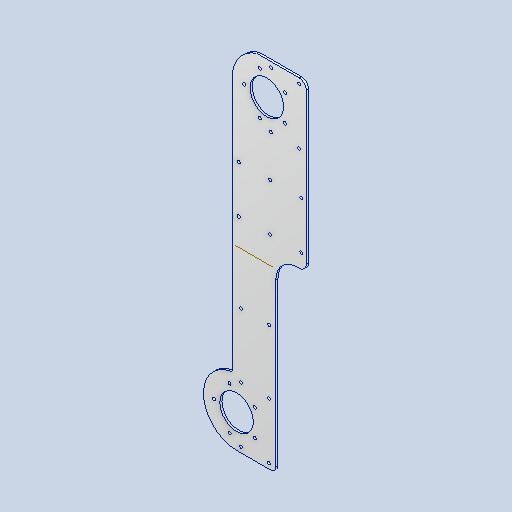
# Autodesk Inventor part: blacha
Saved by Autodesk Inventor 2023 (Build 270158000, 158)
## iProperties
Created: 2023-01-20
Part Number: blacha
Material: Aluminum 6061
Document SubType Name: Modeling
Designer: Kamil
Density: 2.7 g/cm^3
Appearance: Aluminum - Flat
Mass: 107.528 g
Surface Area: 763.261 cm^2
Volume: 107.528 cm^3
Author: Kamil
Autodesk Inventor part; units mm, degrees
ref_plane "YZ Plane" through (0, 0, 0) normal (1, 0, 0) x (0, 1, 0)
ref_plane "XZ Plane" through (0, 0, 0) normal (0, 1, 0) x (-1, 0, 0)
ref_plane "XY Plane" through (0, 0, 0) normal (0, 0, 1) x (1, 0, 0)
sketch "Sketch1" plane through (0, 0, 0) normal (0, 0, 1) x (1, 0, 0)
  circle A0 centre (-40, 69.5) radius 2 projected
  arc A1 (-40, 77) -> (-46, 74) centre (-40, 69.5) ccw projected
  line L0 (-30, 77) -> (-40, 77) projected
  line L1 (-30, 73) -> (-30, 77) projected
  line L2 (-34, 73) -> (-30, 73) projected
  line L3 (-34, 66) -> (-34, 73) projected
  line L4 (-30, 66) -> (-34, 66) projected
  line L5 (-30, 62) -> (-30, 66) projected
  line L6 (-30, 62) -> (-40, 62) projected
  arc A2 (-46, 65) -> (-40, 62) centre (-40, 69.5) ccw projected
  line L7 (-46, 74) -> (-46, 65) projected
  arc A3 (0, 74) -> (-6, 77) centre (-6, 69.5) ccw projected
  line L8 (0, 74) -> (0, 65) projected
  arc A4 (-6, 62) -> (0, 65) centre (-6, 69.5) ccw projected
  line L9 (-6, 62) -> (-16, 62) projected
  line L10 (-16, 66) -> (-16, 62) projected
  line L11 (-12, 66) -> (-16, 66) projected
  line L12 (-12, 73) -> (-12, 66) projected
  line L13 (-16, 73) -> (-12, 73) projected
  line L14 (-16, 77) -> (-16, 73) projected
  line L15 (-6, 77) -> (-16, 77) projected
  circle A5 centre (-6, 69.5) radius 2 projected
  circle A6 centre (-43.375, 22.1232) radius 2 projected
  circle A7 centre (-53.625, 22.1232) radius 2 projected
  circle A8 centre (-38.25, 31) radius 2 projected
  circle A9 centre (-58.75, 31) radius 2 projected
  circle A10 centre (-43.375, 39.8768) radius 2 projected
  arc A11 (-46.014, 25.5393) -> (-48.9684, 25.0183) centre (-48.5, 31) ccw projected
  line L16 (-48.76, 23.8365) -> (-48.9684, 25.0183) projected
  line L17 (-45.8056, 24.3575) -> (-48.76, 23.8365) projected
  line L18 (-46.014, 25.5393) -> (-45.8056, 24.3575) projected
  circle A12 centre (-53.625, 39.8768) radius 2 projected
  circle A13 centre (-48.5, 31) radius 13.4542 projected
  circle A14 centre (-40, -7.5) radius 2 projected
  arc A15 (-40, 0) -> (-46, -3) centre (-40, -7.5) ccw projected
  line L19 (-30, 0) -> (-40, 0) projected
  line L20 (-30, -4) -> (-30, 0) projected
  line L21 (-34, -4) -> (-30, -4) projected
  line L22 (-34, -11) -> (-34, -4) projected
  line L23 (-30, -11) -> (-34, -11) projected
  line L24 (-30, -15) -> (-30, -11) projected
  line L25 (-30, -15) -> (-40, -15) projected
  arc A16 (-46, -12) -> (-40, -15) centre (-40, -7.5) ccw projected
  line L26 (-46, -3) -> (-46, -12) projected
  arc A17 (0, -3) -> (-6, 0) centre (-6, -7.5) ccw projected
  line L27 (0, -3) -> (0, -12) projected
  arc A18 (-6, -15) -> (0, -12) centre (-6, -7.5) ccw projected
  line L28 (-6, -15) -> (-16, -15) projected
  line L29 (-16, -11) -> (-16, -15) projected
  line L30 (-12, -11) -> (-16, -11) projected
  line L31 (-12, -4) -> (-12, -11) projected
  line L32 (-16, -4) -> (-12, -4) projected
  line L33 (-16, 0) -> (-16, -4) projected
  line L34 (-6, 0) -> (-16, 0) projected
  circle A19 centre (-6, -7.5) radius 2 projected
  circle A20 centre (-48.5, 31) radius 27.5 projected
  circle A21 centre (-48.5, 31) radius 24.5
  circle A22 centre (-48.5, 31) radius 19.1667 projected
  circle A23 centre (-48.5, 31) radius 23.3333 projected
  line L35 (-40, -15) -> (-69.5534, -15)
  circle A24 centre (-48.5, 31) radius 46
  line L36 (0, 77) -> (-48.5, 77)
  line L37 (-48.5, 77) -> (-48.5, -15)
  line L38 (-48.5, -15) -> (0, -15)
  line L39 (0, -15) -> (0, 77)
  point P0 (0, 0)
  point P1 (-14.5147, 62)
  point P2 (-16, 63.5538)
  point P3 (-14.5147, 0)
  point P4 (-16, -1.5538)
  point P5 (0, 74)
  point P6 (-6, 77)
  point P7 (-42.4251, 76.5971)
  point P8 (-42.4251, -14.5971)
  point P9 (0, -3)
  constraints: 10 end point, 3 horizontal, 2 parallel, 1 centre point, 1 coincident, 1 perpendicular, 1 point on circle, 1 point on line, 1 tangent, 4 other
extrude "Extrusion1" add sketch "Sketch1" against normal blind 3 contours L0 L1 A24 A1 | A24 L1 L2 L3 L4 L5 L6 A2 L7 A1 | A1 L7 A2 L6 L5 L4 L3 L2 L1 A24 L10 L9 L34 L33 L24 L23 L22 L21 L20 L19 A15 L26 A16 L37 A20 | L36 L14 L13 L12 L11 L10 A24 L1 | L37 A20 A24 | L15 A3 L8 A4 L9 A24 L10 L11 L12 L13 L14 | L37 A21 A20 | A20 L37 A21 | L36 L39 A3 | A16 A24 L24 L25 | A16 L26 A15 L19 L20 L21 L22 L23 L24 A24 | L37 A23 A21 | A21 L37 A23 | L9 A4 L39 A17 L34 A24 | L24 A24 L33 L32 L31 L30 L29 L38 | L29 L30 L31 L32 L33 A24 L34 A17 L27 A18 L28 | A18 L39 L38
sketch "Sketch2" plane through (0, 0, 0) normal (0, 0, 1) x (1, 0, 0)
  line L0 (0, 77) -> (-40, 77) projected
  arc A0 (-40, 77) -> (-42.4251, 76.5971) centre (-40, 69.5) ccw projected
  arc A1 (-42.4251, 76.5971) -> (-42.4251, -14.5971) centre (-48.5, 31) ccw projected
  arc A2 (-42.4251, -14.5971) -> (-40, -15) centre (-40, -7.5) ccw projected
  line L1 (-40, -15) -> (0, -15) projected
  line L2 (0, -15) -> (0, 77) projected
  circle A3 centre (-6, -7.5) radius 2 projected
  line L3 (-14.5147, 62) -> (-16, 62) projected
  line L4 (-16, 62) -> (-16, 63.5538) projected
  arc A4 (-14.5147, 62) -> (-16, 63.5538) centre (-48.5, 31) ccw projected
  circle A5 centre (-6, 69.5) radius 2 projected
  circle A6 centre (-40, -7.5) radius 2 projected
  circle A7 centre (-48.5, 31) radius 23.3333 projected
  circle A8 centre (-40, 69.5) radius 2 projected
  arc A9 (-16, -1.5538) -> (-14.5147, 0) centre (-48.5, 31) ccw projected
  line L5 (-16, -1.5538) -> (-16, 0) projected
  line L6 (-16, 0) -> (-14.5147, 0) projected
  point P0 (0, 0)
extrude "Extrusion2" add sketch "Sketch2" along normal blind 3
extrude "Extrusion3" cut sketch "Sketch2" against normal blind 3
sketch "Sketch3" plane through (0, 0, 3) normal (0, 0, 1) x (1, 0, 0)
  arc A0 (-40, 77) -> (-42.4251, 76.5971) centre (-40, 69.5) ccw projected
  arc A1 (-42.4251, 76.5971) -> (-42.4251, -14.5971) centre (-48.5, 31) ccw projected
  arc A2 (-42.4251, -14.5971) -> (-40, -15) centre (-40, -7.5) ccw projected
  line L0 (-40, -15) -> (0, -15) projected
  line L1 (0, -15) -> (0, 77) projected
  line L2 (0, 77) -> (-40, 77) projected
  circle A3 centre (-6, -7.5) radius 2 projected
  circle A4 centre (-6, 69.5) radius 2 projected
  circle A5 centre (-40, -7.5) radius 2 projected
  circle A6 centre (-40, 69.5) radius 2 projected
  line L3 (-16, 0) -> (-14.5147, 0) projected
  arc A7 (-16, -1.5538) -> (-14.5147, 0) centre (-48.5, 31) ccw projected
  line L4 (-16, -1.5538) -> (-16, 0) projected
  circle A8 centre (-48.5, 31) radius 23.3333 projected
  line L5 (-14.5147, 62) -> (-16, 62) projected
  line L6 (-16, 62) -> (-16, 63.5538) projected
  arc A9 (-14.5147, 62) -> (-16, 63.5538) centre (-48.5, 31) ccw projected
  line L7 (0, -15) -> (0, 77) projected
  arc A10 (-42.4251, 76.5971) -> (-42.4251, -14.5971) centre (-48.5, 31) ccw projected
  line L8 (0, -15) -> (-48.5, -15)
  line L9 (-48.5, -15) -> (-48.5, 31)
  line L10 (-48.5, 31) -> (0, 31)
  line L11 (0, 31) -> (0, -15)
  line L12 (0, 77) -> (-40, 77) projected
  line L13 (0, 77) -> (-48.5, 77)
  line L14 (-48.5, 77) -> (-48.5, 31)
  line L15 (-48.5, 31) -> (0, 31)
  line L16 (0, 31) -> (0, 77)
  line L17 (-7, 271.4196) -> (-7, 337.7)
  line L18 (-39, 271.4196) -> (-39, 337.7)
  line L19 (-48.5, -15) -> (0, -15)
  line L20 (0, -15) -> (0, 420.1653)
  line L21 (0, 420.1653) -> (-48.5, 420.1653)
  line L22 (-48.5, 420.1653) -> (-48.5, -15)
  circle A11 centre (-24.25, 395.9153) radius 24.25
  point P0 (0, 0)
  point P1 (-40, -15)
  point P2 (-48.5, 395.9153)
  point P3 (0, 77)
  point P4 (0, 395.9153)
  constraints: 28 end point, 6 parallel, 3 horizontal, 3 perpendicular, 3 tangent, 2 vertical, 1 centre point, 4 other
extrude "Extrusion4" add sketch "Sketch3" against normal up to surface (3 mm away) contours L13 L22 A11 L20 L2 | A0 A1 L13 | A11 | A1 A2 L8 | L3 A7 L4 | L5 L6 A9
sketch "Sketch4" plane through (0, 0, 3) normal (0, 0, 1) x (1, 0, 0)
  arc A0 (-30.4833, -4.1518) -> (-30.4833, 66.1518) centre (-48.5, 31) ccw projected
  arc A1 (-50.0418, 70.4699) -> (-50.0418, -8.4699) centre (-48.5, 31) ccw projected
  circle A2 centre (-48.5, 31) radius 23.3333 projected
  arc A3 (-50.0418, -8.4699) -> (-43.2432, -5.1587) centre (-49.7295, -0.476) ccw projected
  arc A4 (-38.0441, -4.0108) -> (-43.2432, -5.1587) centre (-40, -7.5) ccw projected
  arc A5 (-38.0441, -4.0108) -> (-30.4833, -4.1518) centre (-34.1323, 2.9676) ccw projected
  arc A6 (-30.4833, 66.1518) -> (-38.0441, 66.0108) centre (-34.1323, 59.0324) ccw projected
  arc A7 (-43.2432, 67.1587) -> (-38.0441, 66.0108) centre (-40, 69.5) ccw projected
  arc A8 (-43.2432, 67.1587) -> (-50.0418, 70.4699) centre (-49.7295, 62.476) ccw projected
  circle A9 centre (-23.0834, 49.4663) radius 3.75 projected
  circle A10 centre (-58.2083, 1.121) radius 3.75 projected
  circle A11 centre (-79.9167, 31) radius 3.75 projected
  circle A12 centre (-23.0834, 12.5337) radius 3.75 projected
  circle A13 centre (-58.2083, 60.879) radius 3.75 projected
  point P0 (0, 0)
  point P1 (-48.5, 31)
  point P2 (-48.5, 31)
  point P3 (-48.5, 31)
  point P4 (-48.5, 31)
extrude "Extrusion5" [suppressed]
sketch "Sketch5" plane through (0, 0, 3) normal (0, 0, 1) x (1, 0, 0)
  circle A0 centre (-23.0834, 49.4663) radius 2.1 projected
  circle A1 centre (-23.0834, 12.5337) radius 2.1 projected
  circle A2 centre (-40, -7.5) radius 2 projected
  circle A3 centre (-58.2083, 1.121) radius 2.1 projected
  circle A4 centre (-79.9167, 31) radius 2.1 projected
  circle A5 centre (-58.2083, 60.879) radius 2.1 projected
  point P0 (0, 0)
extrude "Extrusion6" cut sketch "Sketch5" against normal through all contours A0 | A1 | A3 | A4 | A5
sketch "Sketch6" plane through (0, 0, 3) normal (0, 0, 1) x (1, 0, 0)
  circle A0 centre (-58.2083, 1.121) radius 2.1 projected
  circle A1 centre (-79.9167, 31) radius 2.1 projected
  circle A2 centre (-23.0834, 12.5337) radius 2.1 projected
  circle A3 centre (-58.2083, 60.879) radius 2.1 projected
  circle A4 centre (-23.0834, 49.4663) radius 2.1 projected
  arc A5 (-48.5, 77) -> (-48.5, -15) centre (-48.5, 31) ccw projected
  line L0 (-48.5, -15) -> (0, -15) projected
  line L1 (0, -15) -> (0, 395.9153) projected
  arc A6 (0, 395.9153) -> (-48.5, 395.9153) centre (-24.25, 395.9153) ccw projected
  line L2 (-48.5, 395.9153) -> (-48.5, 77) projected
  circle A7 centre (-6, -7.5) radius 2 projected
  circle A8 centre (-6, 69.5) radius 2 projected
  circle A9 centre (-40, -7.5) radius 2 projected
  circle A10 centre (-40, 69.5) radius 2 projected
  circle A11 centre (-48.5, 31) radius 23.3333 projected
  arc A12 (-6, 135.8558) -> (0, 138.8558) centre (-6, 143.3558) ccw projected
  line L3 (-40, 135.8558) -> (-6, 135.8558) projected
  arc A13 (-46, 138.8558) -> (-40, 135.8558) centre (-40, 143.3558) ccw projected
  line L4 (-46, 138.8558) -> (-46, 147.8558) projected
  arc A14 (-40, 150.8558) -> (-46, 147.8558) centre (-40, 143.3558) ccw projected
  line L5 (-40, 150.8558) -> (-6, 150.8558) projected
  arc A15 (0, 147.8558) -> (-6, 150.8558) centre (-6, 143.3558) ccw projected
  line L6 (0, 138.8558) -> (0, 147.8558) projected
  circle A16 centre (-40, 143.3558) radius 2 projected
  circle A17 centre (-6, 143.3558) radius 2 projected
  point P0 (0, 0)
extrude "Extrusion7" cut sketch "Sketch6" against normal blind 10 contours A16 | A17
sketch "Sketch7" plane through (0, 0, 3) normal (0, 0, 1) x (1, 0, 0)
  arc A0 (-6, -15) -> (0, -12) centre (-6, -7.5) ccw
  line L0 (0, -15) -> (0, 395.9153) projected
  line L1 (-48.5, -15) -> (0, -15) projected
  point P0 (0, 0)
  constraints: 2 point on circle, 1 centre point, 4 other
extrude "Extrusion8" cut sketch "Sketch7" against normal through all
sketch "Sketch8" plane through (0, 0, 3) normal (0, 0, 1) x (1, 0, 0)
  arc A0 (-4, 323.7734) -> (-4, 343.7734) centre (-4, 333.7734) ccw
  arc A1 (-4, 258.1618) -> (-4, 278.1618) centre (-4, 268.1618) ccw
  arc A2 (-42, 278.1618) -> (-42, 258.1618) centre (-42, 268.1618) ccw
  arc A3 (-42, 343.7734) -> (-42, 323.7734) centre (-42, 333.7734) ccw
  circle A4 centre (-48.5, 31) radius 23.3333 projected
  circle A5 centre (-40, 69.5) radius 2 projected
  circle A6 centre (-40, -7.5) radius 2 projected
  circle A7 centre (-6, 69.5) radius 2 projected
  circle A8 centre (-6, -7.5) radius 2 projected
  arc A9 (-6, -15) -> (0, -12) centre (-6, -7.5) ccw projected
  line L0 (0, -12) -> (0, 395.9153) projected
  arc A10 (0, 395.9153) -> (-48.5, 395.9153) centre (-24.25, 395.9153) ccw projected
  line L1 (-48.5, 395.9153) -> (-48.5, 77) projected
  arc A11 (-48.5, 77) -> (-48.5, -15) centre (-48.5, 31) ccw projected
  line L2 (-48.5, -15) -> (-6, -15) projected
  circle A12 centre (-23.0834, 49.4663) radius 2.1 projected
  circle A13 centre (-58.2083, 60.879) radius 2.1 projected
  circle A14 centre (-23.0834, 12.5337) radius 2.1 projected
  circle A15 centre (-79.9167, 31) radius 2.1 projected
  circle A16 centre (-58.2083, 1.121) radius 2.1 projected
  circle A17 centre (-6, 143.3558) radius 2 projected
  circle A18 centre (-40, 143.3558) radius 2 projected
  circle A19 centre (-45.5, 333.7734) radius 2.25
  circle A20 centre (-0.5, 333.7734) radius 2.25
  circle A21 centre (-0.5, 268.1618) radius 2.25
  circle A22 centre (-45.5, 268.1618) radius 2.25
  point P0 (0, 0)
  point P1 (0, 270.3556)
  point P2 (0, 265.9681)
  point P3 (0, 258.9967)
  point P4 (0, 277.327)
  point P5 (-48.5, 260.5625)
  point P6 (-48.5, 275.7612)
  point P7 (-48.5, 326.174)
  point P8 (-48.5, 341.3727)
  point P9 (0, 335.9671)
  point P10 (0, 331.5796)
  point P11 (0, 324.6082)
  point P12 (0, 342.9385)
  constraints: 8 centre point, 8 point on circle, 24 other
extrude "Extrusion9" add sketch "Sketch8" against normal up to surface (3 mm away) contours L0 A20 A0 | A1 L0 A21 | L1 A3 | L1 A2
extrude "Extrusion10" cut sketch "Sketch8" against normal through all contours A20 L0 | A21 L0 | L0 A21 | A19 | A22 picked at (-0.9113, 333.6839)
sketch "Sketch9" plane through (0, 0, 3) normal (0, 0, 1) x (1, 0, 0)
  circle A0 centre (-45.5, 268.1618) radius 2.25 projected
  circle A1 centre (-45.5, 333.7734) radius 2.25 projected
  circle A2 centre (-0.5, 333.7734) radius 2.25 projected
  circle A3 centre (-0.5, 268.1618) radius 2.25 projected
  circle A4 centre (-48.5, 31) radius 23.3333 projected
  circle A5 centre (-40, 69.5) radius 2 projected
  circle A6 centre (-40, -7.5) radius 2 projected
  circle A7 centre (-6, 69.5) radius 2 projected
  circle A8 centre (-6, -7.5) radius 2 projected
  arc A9 (0, 324.6082) -> (0, 342.9385) centre (-4, 333.7734) ccw projected
  line L0 (0, 342.9385) -> (0, 395.9153) projected
  arc A10 (0, 395.9153) -> (-48.5, 395.9153) centre (-24.25, 395.9153) ccw projected
  line L1 (-48.5, 395.9153) -> (-48.5, 341.3727) projected
  arc A11 (-48.5, 341.3727) -> (-48.5, 326.174) centre (-42, 333.7734) ccw projected
  line L2 (-48.5, 326.174) -> (-48.5, 275.7612) projected
  arc A12 (-48.5, 275.7612) -> (-48.5, 260.5625) centre (-42, 268.1618) ccw projected
  line L3 (-48.5, 260.5625) -> (-48.5, 77) projected
  arc A13 (-48.5, 77) -> (-48.5, -15) centre (-48.5, 31) ccw projected
  line L4 (-48.5, -15) -> (-6, -15) projected
  arc A14 (-6, -15) -> (0, -12) centre (-6, -7.5) ccw projected
  line L5 (0, -12) -> (0, 258.9967) projected
  arc A15 (0, 258.9967) -> (0, 277.327) centre (-4, 268.1618) ccw projected
  line L6 (0, 277.327) -> (0, 324.6082) projected
  circle A16 centre (-23.0834, 49.4663) radius 2.1 projected
  circle A17 centre (-58.2083, 60.879) radius 2.1 projected
  circle A18 centre (-23.0834, 12.5337) radius 2.1 projected
  circle A19 centre (-79.9167, 31) radius 2.1 projected
  circle A20 centre (-58.2083, 1.121) radius 2.1 projected
  circle A21 centre (-6, 143.3558) radius 2 projected
  circle A22 centre (-40, 143.3558) radius 2 projected
  line L7 (6, 333.7734) -> (6, 443.3902)
  circle A23 centre (-24.25, 395.9153) radius 30.25
  line L8 (-54.5, 395.9153) -> (-54.5, 76.607)
  arc A24 (-48.5, 77) -> (-48.5, -15) centre (-48.5, 31) ccw projected
  line L9 (6, 333.7734) -> (6, -15)
  arc A25 (0, 324.6082) -> (0, 342.9385) centre (-4, 333.7734) ccw projected
  line L10 (-48.5, -15) -> (-6, -15) projected
  line L11 (6, -15) -> (-6, -15)
  point P0 (0, 0)
  point P1 (6, 395.9153)
  point P2 (6, 268.1618)
  constraints: 8 end point, 4 vertical, 2 point on circle, 1 coincident, 1 perpendicular, 1 tangent, 3 other
extrude "Extrusion11" add sketch "Sketch9" against normal up to surface (3 mm away) contours A5 | A6 | A7 | A8 | A9 L9 A15 L6 | A9 L0 A23 L7 | A23 L0 A10 L1 | L9 L11 A14 L5 A15 | A23 L1 A11 L2 A12 L3 A13 L8 | A21 | A22 picked at (1.094, 385.7102)
sketch "Sketch10" plane through (0, 0, 0) normal (0, 0, -1) x (-1, 0, 0)
  circle A0 centre (3.5, -7.7) radius 2
  circle A1 centre (42.5, -7.7) radius 2
  circle A2 centre (42.5, 69.94) radius 2
  circle A3 centre (3.5, 69.94) radius 2
  circle A4 centre (3.5, 158.6736) radius 2
  circle A5 centre (42.5, 158.6736) radius 2
  point P0 (0, 0)
  constraints: 6 centre point, 12 other
extrude "Extrusion12" cut sketch "Sketch10" against normal up to surface (3 mm away)
fillet "Fillet1" radius 7 1 edges at (6, -15, 1.5)
sketch "Sketch11" plane through (0, 0, 0) normal (0, 0, -1) x (-1, 0, 0)
  arc A0 (-6, -8) -> (1, -15) centre (1, -8) ccw projected
  line L0 (48.5, -15) -> (1, -15) projected
  arc A1 (48.5, -15) -> (54.5, 76.607) centre (48.5, 31) ccw projected
  line L1 (54.5, 76.607) -> (54.5, 395.9153) projected
  arc A2 (54.5, 395.9153) -> (-6, 395.9153) centre (24.25, 395.9153) ccw projected
  line L2 (-6, 395.9153) -> (-6, -8) projected
  circle A3 centre (3.5, 69.94) radius 2 projected
  circle A4 centre (3.5, -7.7) radius 2 projected
  circle A5 centre (42.5, 158.6736) radius 2 projected
  circle A6 centre (42.5, 69.94) radius 2 projected
  circle A7 centre (42.5, -7.7) radius 2 projected
  circle A8 centre (3.5, 158.6736) radius 2 projected
  circle A9 centre (0.5, 268.1618) radius 2.25 projected
  circle A10 centre (0.5, 333.7734) radius 2.25 projected
  circle A11 centre (45.5, 268.1618) radius 2.25 projected
  circle A12 centre (45.5, 333.7734) radius 2.25 projected
  circle A13 centre (58.2083, 1.121) radius 2.1 projected
  circle A14 centre (79.9167, 31) radius 2.1 projected
  circle A15 centre (23.0834, 12.5337) radius 2.1 projected
  circle A16 centre (58.2083, 60.879) radius 2.1 projected
  circle A17 centre (23.0834, 49.4663) radius 2.1 projected
  circle A18 centre (48.5, 31) radius 23.3333 projected
  arc A19 (54.5, 395.9153) -> (-6, 395.9153) centre (24.25, 395.9153) ccw projected
  line L3 (54.5, 395.9153) -> (88.029, 429.4443)
  line L4 (54.5, 395.9153) -> (101.9172, 395.9153) construction
  line L5 (-6, 395.9153) -> (50.7056, 452.6209)
  line L6 (-6, 395.9153) -> (74.1938, 395.9153) construction
  line L7 (54.5, 395.9153) -> (99.5, 395.9153)
  line L8 (54.5, 395.9153) -> (99.5, 440.9153)
  line L9 (99.5, 440.9153) -> (56.72, 483.6952)
  line L10 (56.72, 483.6952) -> (-6, 418.4153)
  line L11 (-6, 418.4153) -> (-6, 395.9153)
  circle A20 centre (78.11, 462.3053) radius 30.25
  point P0 (0, 0)
  dimension "d25" = 45
  dimension "d26" = 45
  dimension "d27" = 45
  dimension "d28" = 60.5
  constraints: 18 end point, 2 equal length, 2 horizontal, 2 point on line, 1 midpoint, 1 point on circle, 3 other
  measures "d25" angle of L4 L3
  measures "d26" angle of L6 L5
  measures "d27" distance of L1.end L7.end
  measures "d28" distance of L9.start L9.end
extrude "Extrusion13" add sketch "Sketch11" against normal blind 3 contours L11 L10 A20 L5 A2 | L5 A20 L8 L3 A2 | A20 L10 L9 | L9 A20
fillet "Fillet2" radius 2 1 edges at (-54.5, 76.607, 1.5)
fillet "Fillet3" radius 15 2 edges at (-54.5, 395.9153, 1.5) (6, 418.4153, 1.5)
sketch "Sketch12" plane through (0, 0, 0) normal (0, 0, -1) x (-1, 0, 0)
  arc A0 (-1.8166, 422.7695) -> (-6, 412.3771) centre (9, 412.3771) ccw projected
  line L0 (-6, 412.3771) -> (-6, -8) projected
  arc A1 (-6, -8) -> (1, -15) centre (1, -8) ccw projected
  line L1 (48.5, -15) -> (1, -15) projected
  arc A2 (48.5, -15) -> (56.1667, 76.3566) centre (48.5, 31) ccw projected
  arc A3 (54.5, 78.3286) -> (56.1667, 76.3566) centre (56.5, 78.3286) ccw projected
  line L2 (54.5, 78.3286) -> (54.5, 389.7021) projected
  arc A4 (58.8934, 400.3087) -> (54.5, 389.7021) centre (69.5, 389.7021) ccw projected
  line L3 (58.8934, 400.3087) -> (99.5, 440.9153) projected
  arc A5 (99.5, 440.9153) -> (56.72, 483.6952) centre (78.11, 462.3053) ccw projected
  line L4 (56.72, 483.6952) -> (-1.8166, 422.7695) projected
  circle A6 centre (3.5, 69.94) radius 2 projected
  circle A7 centre (3.5, -7.7) radius 2 projected
  circle A8 centre (42.5, 158.6736) radius 2 projected
  circle A9 centre (42.5, 69.94) radius 2 projected
  circle A10 centre (42.5, -7.7) radius 2 projected
  circle A11 centre (3.5, 158.6736) radius 2 projected
  circle A12 centre (0.5, 268.1618) radius 2.25 projected
  circle A13 centre (0.5, 333.7734) radius 2.25 projected
  circle A14 centre (45.5, 268.1618) radius 2.25 projected
  circle A15 centre (45.5, 333.7734) radius 2.25 projected
  circle A16 centre (58.2083, 1.121) radius 2.1 projected
  circle A17 centre (79.9167, 31) radius 2.1 projected
  circle A18 centre (23.0834, 12.5337) radius 2.1 projected
  circle A19 centre (58.2083, 60.879) radius 2.1 projected
  circle A20 centre (23.0834, 49.4663) radius 2.1 projected
  circle A21 centre (48.5, 31) radius 23.3333 projected
  circle A22 centre (69.5, 389.7021) radius 15
  circle A23 centre (9, 412.3771) radius 15
  circle A24 centre (78.11, 462.3053) radius 30.25
  arc A25 (58.8934, 400.3087) -> (54.5, 389.7021) centre (69.5, 389.7021) ccw projected
  circle A26 centre (9, 438.3771) radius 15
  circle A27 centre (69.5, 415.7021) radius 15
  arc A28 (99.5, 440.9153) -> (56.72, 483.6952) centre (78.11, 462.3053) ccw projected
  circle A29 centre (78.11, 488.3053) radius 30.25
  line L5 (45.5903, 413.0056) -> (126.2589, 493.6742)
  line L6 (-11.4322, 438.76) -> (94.3242, 548.8486)
  line L7 (54.5, 389.7021) -> (54.5, 415.7021)
  arc A30 (-1.8166, 422.7695) -> (-6, 412.3771) centre (9, 412.3771) ccw projected
  line L8 (-6, 412.3771) -> (-6, 438.3771)
  point P0 (0, 0)
  point P1 (-1.8173, 448.7687)
  point P2 (-6, 412.3771)
  point P3 (55.8819, 482.8229)
  point P4 (56.72, 483.6952)
  point P5 (105.4242, 475.3053)
  point P6 (56.2951, 509.2617)
  point P7 (106.1759, 473.5911)
  point P8 (58.8934, 426.3087)
  constraints: 8 end point, 5 tangent, 4 centre point, 3 coincident, 1 concentric, 1 parallel, 1 point on circle, 1 vertical, 9 other
extrude "Extrusion14" add sketch "Sketch12" against normal up to surface (3 mm away) contours A0 L8 A26 L4 | A26 L4 | A26 L6 A29 L4 | A29 A5 A24 L4 picked at (80.5899, 500.9461)
extrude "Extrusion15" cut sketch "Sketch12" against normal through all contours L5 A5 A24 | A24 L3 A27 L5 | A27 L3 | L7 A27 L3 A4
sketch "Sketch13" plane through (0, 0, 0) normal (0, 0, -1) x (-1, 0, 0)
  line L0 (58.8934, 426.3087) -> (106.1759, 473.5911) projected
  arc A0 (106.1759, 473.5911) -> (105.4242, 475.3053) centre (78.11, 462.3053) ccw projected
  arc A1 (105.4242, 475.3053) -> (56.2951, 509.2617) centre (78.11, 488.3053) ccw projected
  line L1 (56.2951, 509.2617) -> (-1.8173, 448.7687) projected
  arc A2 (-1.8173, 448.7687) -> (-6, 438.3771) centre (9, 438.3771) ccw projected
  line L2 (-6, 438.3771) -> (-6, -8) projected
  arc A3 (-6, -8) -> (1, -15) centre (1, -8) ccw projected
  line L3 (48.5, -15) -> (1, -15) projected
  arc A4 (48.5, -15) -> (56.1667, 76.3566) centre (48.5, 31) ccw projected
  arc A5 (54.5, 78.3286) -> (56.1667, 76.3566) centre (56.5, 78.3286) ccw projected
  line L4 (54.5, 78.3286) -> (54.5, 415.7021) projected
  arc A6 (58.8934, 426.3087) -> (54.5, 415.7021) centre (69.5, 415.7021) ccw projected
  arc A7 (56.72, 483.6952) -> (55.8819, 482.8229) centre (78.11, 462.3053) ccw projected
  line L5 (56.72, 483.6952) -> (55.8819, 482.8229) projected
  circle A8 centre (3.5, 69.94) radius 2 projected
  circle A9 centre (3.5, -7.7) radius 2 projected
  circle A10 centre (42.5, 158.6736) radius 2 projected
  circle A11 centre (42.5, 69.94) radius 2 projected
  circle A12 centre (42.5, -7.7) radius 2 projected
  circle A13 centre (3.5, 158.6736) radius 2 projected
  circle A14 centre (0.5, 268.1618) radius 2.25 projected
  circle A15 centre (0.5, 333.7734) radius 2.25 projected
  circle A16 centre (45.5, 268.1618) radius 2.25 projected
  circle A17 centre (45.5, 333.7734) radius 2.25 projected
  circle A18 centre (58.2083, 1.121) radius 2.1 projected
  circle A19 centre (79.9167, 31) radius 2.1 projected
  circle A20 centre (23.0834, 12.5337) radius 2.1 projected
  circle A21 centre (58.2083, 60.879) radius 2.1 projected
  circle A22 centre (23.0834, 49.4663) radius 2.1 projected
  circle A23 centre (48.5, 31) radius 23.3333 projected
  line L6 (54.5, 78.3286) -> (54.5, 415.7021) projected
  line L7 (54.5, 415.7021) -> (54.5, 390.7021)
  line L8 (54.5, 390.7021) -> (-6, 390.7021)
  line L9 (-6, 438.3771) -> (-6, -8) projected
  point P0 (0, 0)
  point P1 (-6, 390.7021)
  dimension "d41" = 25
  constraints: 4 end point, 2 point on line, 1 perpendicular
  measures "d41" distance of L4.end L7.end
extrude "Extrusion16" add sketch "Sketch13" along normal blind 30.35 contours A6 L4 L8 L2 A2 L1 A1 A0 L0
sketch "Sketch14" plane through (0, 0, 3) normal (0, 0, 1) x (1, 0, 0)
  circle A0 centre (-58.2083, 1.121) radius 2.1 projected
  circle A1 centre (-79.9167, 31) radius 2.1 projected
  circle A2 centre (-23.0834, 12.5337) radius 2.1 projected
  circle A3 centre (-58.2083, 60.879) radius 2.1 projected
  circle A4 centre (-23.0834, 49.4663) radius 2.1 projected
  line L0 (-106.1759, 473.5911) -> (-58.8934, 426.3087) projected
  arc A5 (-54.5, 415.7021) -> (-58.8934, 426.3087) centre (-69.5, 415.7021) ccw projected
  line L1 (-54.5, 415.7021) -> (-54.5, 78.3286) projected
  arc A6 (-56.1667, 76.3566) -> (-54.5, 78.3286) centre (-56.5, 78.3286) ccw projected
  arc A7 (-56.1667, 76.3566) -> (-48.5, -15) centre (-48.5, 31) ccw projected
  line L2 (-48.5, -15) -> (-1, -15) projected
  arc A8 (-1, -15) -> (6, -8) centre (-1, -8) ccw projected
  line L3 (6, 438.3771) -> (6, -8) projected
  arc A9 (6, 438.3771) -> (1.8173, 448.7687) centre (-9, 438.3771) ccw projected
  line L4 (-56.2951, 509.2617) -> (1.8173, 448.7687) projected
  arc A10 (-56.2951, 509.2617) -> (-105.4242, 475.3053) centre (-78.11, 488.3053) ccw projected
  arc A11 (-105.4242, 475.3053) -> (-106.1759, 473.5911) centre (-78.11, 462.3053) ccw projected
  circle A12 centre (-48.5, 31) radius 23.3333 projected
  circle A13 centre (-0.5, 268.1618) radius 2.25 projected
  circle A14 centre (-0.5, 333.7734) radius 2.25 projected
  circle A15 centre (-45.5, 333.7734) radius 2.25 projected
  circle A16 centre (-45.5, 268.1618) radius 2.25 projected
  circle A17 centre (-3.5, 158.6736) radius 2 projected
  circle A18 centre (-42.5, -7.7) radius 2 projected
  circle A19 centre (-42.5, 69.94) radius 2 projected
  circle A20 centre (-42.5, 158.6736) radius 2 projected
  circle A21 centre (-3.5, -7.7) radius 2 projected
  circle A22 centre (-3.5, 69.94) radius 2 projected
  line L5 (-55.8819, 482.8229) -> (-56.72, 483.6952) projected
  arc A23 (-55.8819, 482.8229) -> (-56.72, 483.6952) centre (-78.11, 462.3053) ccw projected
  line L6 (6, 438.3771) -> (6, 390.7021) projected
  line L7 (6, 390.7021) -> (-54.5, 390.7021) projected
  line L8 (-54.5, 390.7021) -> (-54.5, 415.7021) projected
  arc A24 (-54.5, 415.7021) -> (-58.8934, 426.3087) centre (-69.5, 415.7021) ccw projected
  line L9 (-58.8934, 426.3087) -> (-106.1759, 473.5911) projected
  arc A25 (-105.4242, 475.3053) -> (-106.1759, 473.5911) centre (-78.11, 462.3053) ccw projected
  arc A26 (-56.2951, 509.2617) -> (-105.4242, 475.3053) centre (-78.11, 488.3053) ccw projected
  line L10 (-56.2951, 509.2617) -> (1.8173, 448.7687) projected
  arc A27 (6, 438.3771) -> (1.8173, 448.7687) centre (-9, 438.3771) ccw projected
  line L11 (-56.72, 483.6952) -> (-55.8819, 482.8229) projected
  arc A28 (-55.8819, 482.8229) -> (-56.72, 483.6952) centre (-78.11, 462.3053) ccw projected
  line L12 (6, 438.3771) -> (6, 390.7021) projected
  line L13 (-54.5, 390.7021) -> (6, 390.7021)
  line L14 (6, 390.7021) -> (6, 393.7021)
  line L15 (6, 393.7021) -> (-54.5, 393.7021)
  line L16 (-54.5, 393.7021) -> (-54.5, 390.7021)
  point P0 (0, 0)
  dimension "d44" = 3
  constraints: 8 end point, 2 parallel, 1 horizontal, 1 perpendicular, 1 point on line
  measures "d44" distance of L14.end L13.end
extrude "Extrusion17" cut sketch "Sketch14" against normal blind 30.35 contours A11 A10 L4 A9 L3 L15 L1 A5 L0
fillet "Fillet4" radius 3 4 edges at (-24.25, 390.7021, -30.35) (-24.25, 393.7021, 3) (-24.25, 390.7021, 0) (-24.25, 393.7021, -27.35)
sketch "Sketch15" plane through (0, 0, 3) normal (0, 0, 1) x (1, 0, 0)
  circle A0 centre (-58.2083, 1.121) radius 2.1 projected
  circle A1 centre (-79.9167, 31) radius 2.1 projected
  circle A2 centre (-23.0834, 12.5337) radius 2.1 projected
  circle A3 centre (-58.2083, 60.879) radius 2.1 projected
  circle A4 centre (-23.0834, 49.4663) radius 2.1 projected
  line L0 (-54.5, 390.7021) -> (6, 390.7021) projected
  line L1 (-54.5, 390.7021) -> (-54.5, 78.3286) projected
  arc A5 (-56.1667, 76.3566) -> (-54.5, 78.3286) centre (-56.5, 78.3286) ccw projected
  arc A6 (-56.1667, 76.3566) -> (-48.5, -15) centre (-48.5, 31) ccw projected
  line L2 (-48.5, -15) -> (-1, -15) projected
  arc A7 (-1, -15) -> (6, -8) centre (-1, -8) ccw projected
  line L3 (6, 390.7021) -> (6, -8) projected
  circle A8 centre (-48.5, 31) radius 23.3333 projected
  circle A9 centre (-0.5, 268.1618) radius 2.25 projected
  circle A10 centre (-0.5, 333.7734) radius 2.25 projected
  circle A11 centre (-45.5, 333.7734) radius 2.25 projected
  circle A12 centre (-45.5, 268.1618) radius 2.25 projected
  circle A13 centre (-3.5, 158.6736) radius 2 projected
  circle A14 centre (-42.5, -7.7) radius 2 projected
  circle A15 centre (-42.5, 69.94) radius 2 projected
  circle A16 centre (-42.5, 158.6736) radius 2 projected
  circle A17 centre (-3.5, -7.7) radius 2 projected
  circle A18 centre (-3.5, 69.94) radius 2 projected
  arc A19 (-56.1667, 76.3566) -> (-48.5, -15) centre (-48.5, 31) ccw projected
  line L4 (6, 390.7021) -> (-54.5, 390.7021) projected
  line L5 (6, 390.7021) -> (-168.056, 390.7021)
  line L6 (-168.056, 390.7021) -> (-168.056, 602.0658)
  line L7 (-168.056, 602.0658) -> (6, 602.0658)
  line L8 (6, 602.0658) -> (6, 390.7021)
  point P0 (0, 0)
  constraints: 8 end point, 2 parallel, 1 horizontal, 1 perpendicular
extrude "Extrusion18" cut sketch "Sketch15" against normal through all contours L5 L6 L7 L8 L0
sketch "Sketch16" plane through (0, 0, 3) normal (0, 0, 1) x (1, 0, 0)
  circle A0 centre (-48.5, 31) radius 23.3333 projected
  line L0 (-48.5, 31) -> (-48.5, 431)
  line L1 (-54.5, 390.7021) -> (-54.5, 78.3286) projected
  circle A1 centre (-48.5, 431) radius 23.3333
  circle A2 centre (-58.2083, 1.121) radius 2.1 projected
  circle A3 centre (-79.9167, 31) radius 2.1 projected
  circle A4 centre (-23.0834, 12.5337) radius 2.1 projected
  circle A5 centre (-58.2083, 60.879) radius 2.1 projected
  circle A6 centre (-23.0834, 49.4663) radius 2.1 projected
  line L2 (-54.5, 390.7021) -> (6, 390.7021) projected
  line L3 (-54.5, 390.7021) -> (-54.5, 78.3286) projected
  arc A7 (-56.1667, 76.3566) -> (-54.5, 78.3286) centre (-56.5, 78.3286) ccw projected
  arc A8 (-56.1667, 76.3566) -> (-48.5, -15) centre (-48.5, 31) ccw projected
  line L4 (-48.5, -15) -> (-1, -15) projected
  arc A9 (-1, -15) -> (6, -8) centre (-1, -8) ccw projected
  line L5 (6, 390.7021) -> (6, -8) projected
  circle A10 centre (-48.5, 31) radius 23.3333 projected
  circle A11 centre (-0.5, 268.1618) radius 2.25 projected
  circle A12 centre (-0.5, 333.7734) radius 2.25 projected
  circle A13 centre (-45.5, 333.7734) radius 2.25 projected
  circle A14 centre (-45.5, 268.1618) radius 2.25 projected
  circle A15 centre (-3.5, 158.6736) radius 2 projected
  circle A16 centre (-42.5, -7.7) radius 2 projected
  circle A17 centre (-42.5, 69.94) radius 2 projected
  circle A18 centre (-42.5, 158.6736) radius 2 projected
  circle A19 centre (-3.5, -7.7) radius 2 projected
  circle A20 centre (-3.5, 69.94) radius 2 projected
  line L6 (-48.5, 231) -> (-140.0834, 231)
  circle A21 centre (-48.5, 431) radius 23.3333
  line L7 (-48.5, 431) -> (-48.5, 31)
  line L8 (-54.5, 71.2979) -> (-54.5, 383.6714)
  circle A22 centre (-58.2083, 460.879) radius 2.1
  circle A23 centre (-79.9167, 431) radius 2.1
  circle A24 centre (-23.0834, 449.4663) radius 2.1
  circle A25 centre (-58.2083, 401.121) radius 2.1
  circle A26 centre (-23.0834, 412.5337) radius 2.1
  line L9 (-54.5, 71.2979) -> (-54.5, 383.6714)
  arc A27 (-54.5, 383.6714) -> (-56.1667, 385.6434) centre (-56.5, 383.6714) ccw
  arc A28 (-48.5, 477) -> (-56.1667, 385.6434) centre (-48.5, 431) ccw
  line L10 (-48.5, 477) -> (-1, 477)
  arc A29 (6, 470) -> (-1, 477) centre (-1, 470) ccw
  line L11 (6, 71.2979) -> (6, 470)
  circle A30 centre (-48.5, 431) radius 23.3333
  circle A31 centre (-3.5, 303.3264) radius 2
  circle A32 centre (-42.5, 469.7) radius 2
  circle A33 centre (-42.5, 392.06) radius 2
  circle A34 centre (-42.5, 303.3264) radius 2
  circle A35 centre (-3.5, 469.7) radius 2
  circle A36 centre (-3.5, 392.06) radius 2
  point P0 (0, 0)
  point P1 (0, 462)
  point P2 (-43.9684, 390.7021)
  point P3 (-41.0316, 390.7021)
  point P4 (-4.9684, 390.7021)
  point P5 (-2.0316, 390.7021)
  dimension "d51" = 400
  constraints: 27 symmetric about line, 17 centre point, 14 end point, 6 point on circle, 1 coincident, 1 horizontal, 1 midpoint, 1 parallel, 16 other
  measures "d51" distance of L0.start L0.end
extrude "Extrusion19" add sketch "Sketch16" against normal up to surface (3 mm away) contours L2 L1 A27 A28 L10 A29 L11 A36 A33
sketch "Sketch17" plane through (6, -8, 0) normal (1, 0, 0) x (0, 0, -1)
  line L0 (3, 398.7021) -> (0, 398.7021) projected
  line L1 (0, 478) -> (0, 398.7021) projected
  line L2 (-3, 478) -> (0, 478) projected
  line L3 (-3, 478) -> (-3, 0) projected
  line L4 (0, 0) -> (-3, 0) projected
  line L5 (0, 395.7021) -> (0, 0) projected
  arc A0 (3, 398.7021) -> (0, 395.7021) centre (3, 395.7021) ccw projected
  line L6 (0, 478) -> (0, 398.7021) projected
  line L7 (0, 398.7021) -> (0, 395.7021)
  arc A1 (3, 398.7021) -> (0, 395.7021) centre (3, 395.7021) ccw projected
  point P0 (0, 8)
  constraints: 2 end point, 1 point on circle, 1 vertical
extrude "Extrusion20" cut sketch "Sketch17" against normal through all contours A0 L7 L0
ref_plane "Work Plane1" through (-48.5, 231, 0) normal (0, -1, 0) x (1, 0, 0)
sketch "Sketch18" plane through (0, 0, 0) normal (0, 0, -1) x (-1, 0, 0)
  line L0 (7, 279.9) -> (7, 230.5)
  line L1 (7, 280.4196) -> (7, 346.7)
  line L2 (39, 280.4196) -> (39, 346.7)
  arc A0 (4.9684, 390.7021) -> (2.0316, 390.7021) centre (3.5, 392.06) ccw projected
  line L3 (2.0316, 390.7021) -> (4.9684, 390.7021) projected
  line L4 (-6, 470) -> (-6, -8) projected
  arc A1 (-6, -8) -> (1, -15) centre (1, -8) ccw projected
  line L5 (48.5, -15) -> (1, -15) projected
  arc A2 (48.5, -15) -> (56.1667, 76.3566) centre (48.5, 31) ccw projected
  arc A3 (54.5, 78.3286) -> (56.1667, 76.3566) centre (56.5, 78.3286) ccw projected
  line L6 (54.5, 78.3286) -> (54.5, 383.6714) projected
  arc A4 (56.1667, 385.6434) -> (54.5, 383.6714) centre (56.5, 383.6714) ccw projected
  arc A5 (56.1667, 385.6434) -> (48.5, 477) centre (48.5, 431) ccw projected
  line L7 (48.5, 477) -> (1, 477) projected
  arc A6 (1, 477) -> (-6, 470) centre (1, 470) ccw projected
  circle A7 centre (48.5, 431) radius 23.3333 projected
  circle A8 centre (42.5, 469.7) radius 2 projected
  circle A9 centre (3.5, 469.7) radius 2 projected
  circle A10 centre (58.2083, 460.879) radius 2.1 projected
  circle A11 centre (23.0834, 449.4663) radius 2.1 projected
  circle A12 centre (79.9167, 431) radius 2.1 projected
  circle A13 centre (23.0834, 412.5337) radius 2.1 projected
  circle A14 centre (58.2083, 401.121) radius 2.1 projected
  circle A15 centre (3.5, 69.94) radius 2 projected
  circle A16 centre (3.5, -7.7) radius 2 projected
  circle A17 centre (42.5, 158.6736) radius 2 projected
  circle A18 centre (42.5, 69.94) radius 2 projected
  circle A19 centre (42.5, -7.7) radius 2 projected
  circle A20 centre (3.5, 158.6736) radius 2 projected
  circle A21 centre (0.5, 268.1618) radius 2.25 projected
  circle A22 centre (0.5, 333.7734) radius 2.25 projected
  circle A23 centre (45.5, 268.1618) radius 2.25 projected
  circle A24 centre (45.5, 333.7734) radius 2.25 projected
  circle A25 centre (58.2083, 1.121) radius 2.1 projected
  circle A26 centre (79.9167, 31) radius 2.1 projected
  circle A27 centre (23.0834, 12.5337) radius 2.1 projected
  circle A28 centre (58.2083, 60.879) radius 2.1 projected
  circle A29 centre (23.0834, 49.4663) radius 2.1 projected
  circle A30 centre (48.5, 31) radius 23.3333 projected
  line L8 (41.0316, 390.7021) -> (43.9684, 390.7021) projected
  arc A31 (43.9684, 390.7021) -> (41.0316, 390.7021) centre (42.5, 392.06) ccw projected
  line L9 (7, 285.9302) -> (-6, 285.9302)
  line L10 (39, 285.9302) -> (54.5, 285.9302)
  line L11 (54.5, 383.6714) -> (54.5, 78.3286) projected
  line L12 (39, 285.9302) -> (49, 285.9302)
  line L13 (49, 285.9302) -> (49, 345.4465)
  line L14 (49, 345.4465) -> (39, 345.4465)
  line L15 (39, 345.4465) -> (39, 285.9302)
  line L16 (49, 345.4465) -> (81, 345.4465)
  line L17 (81, 345.4465) -> (81, 285.9302)
  line L18 (81, 285.9302) -> (49, 285.9302)
  line L19 (49, 285.9302) -> (49, 345.4465)
  line L20 (7, 230.5) -> (-3, 230.5)
  line L21 (-3, 230.5) -> (-3, 345.4465)
  line L22 (-3, 345.4465) -> (7, 345.4465)
  line L23 (7, 345.4465) -> (7, 230.5)
  line L24 (-3, 345.4465) -> (-35, 345.4465)
  line L25 (-35, 345.4465) -> (-35, 247.7791)
  line L26 (-35, 247.7791) -> (-3, 247.7791)
  line L27 (-3, 247.7791) -> (-3, 345.4465)
  line L28 (-35, 247.7791) -> (-50.5, 247.7791)
  line L29 (-50.5, 247.7791) -> (-50.5, 345.4465)
  line L30 (-50.5, 345.4465) -> (-35, 345.4465)
  line L31 (-35, 345.4465) -> (-35, 247.7791)
  line L32 (-19, 345.4465) -> (-19, 501.6189)
  line L33 (39, 285.9302) -> (7, 285.9302)
  line L34 (23, 285.9302) -> (23, -113.535)
  line L35 (48.5, 31) -> (23, 31)
  line L36 (-19, 431) -> (6.5, 431)
  circle A32 centre (6.5, 431) radius 23.3333
  arc A33 (56.1667, 385.6434) -> (54.5, 383.6714) centre (56.5, 383.6714) ccw projected
  line L37 (-50.5, 345.4465) -> (-50.5, 477)
  line L38 (-50.5, 477) -> (1, 477)
  circle A34 centre (3.5, -7.7) radius 2 projected
  line L39 (3.5, -7.7) -> (23, -7.7)
  line L40 (-19, 477) -> (-38.5, 477)
  line L41 (-38.5, 477) -> (-38.5, 345.4465)
  line L42 (-38.5, 345.4465) -> (-19, 345.4465)
  line L43 (-19, 345.4465) -> (-19, 477)
  line L44 (-6, 470) -> (-6, -8) projected
  line L45 (-50.5, 477) -> (-6, 477)
  line L46 (-6, 477) -> (-6, 469.7)
  line L47 (-6, 469.7) -> (-50.5, 469.7)
  line L48 (-50.5, 469.7) -> (-50.5, 477)
  circle A35 centre (-38.5, 469.7) radius 2
  line L49 (-38.5, 469.7) -> (0.5, 469.7)
  circle A36 centre (0.5, 469.7) radius 2
  line L50 (54.5, 383.6714) -> (54.5, 504.9816)
  circle A37 centre (6.5, 431) radius 48
  line L51 (0.5, 469.7) -> (-38.5, 469.7)
  line L52 (-38.5, 469.7) -> (-38.5, 392.06)
  line L53 (-38.5, 392.06) -> (0.5, 392.06)
  line L54 (0.5, 392.06) -> (0.5, 469.7)
  circle A38 centre (0.5, 392.06) radius 2
  circle A39 centre (-38.5, 392.06) radius 2
  point P0 (0, 0)
  point P1 (-6, 247.7791)
  point P2 (20.9909, 412.7118)
  point P3 (23.1305, 414.6332)
  point P4 (27.5, 420.8292)
  point P5 (27.5, 441.1708)
  point P6 (23.1305, 447.3668)
  point P7 (20.9909, 449.2882)
  point P8 (54.5, 408.4513)
  point P9 (20.2113, 477)
  point P10 (48.4471, 454.3333)
  point P11 (2, 471.0229)
  point P12 (2, 468.3771)
  point P13 (2, 393.3829)
  point P14 (2, 390.7371)
  point P15 (54.5, 431)
  dimension "d57" = 10
  dimension "d58" = 32
  dimension "d59" = 10
  dimension "d60" = 32
  dimension "d61" = 15.5
  dimension "d62" = 25.5
  dimension "d64" = 19.5
  dimension "d65" = 19.5
  dimension "d66" = 7.3
  dimension "d67" = 4
  dimension "d68" = 39
  dimension "d69" = 4
  dimension "d70" = 4
  dimension "d71" = 4
  constraints: 94 end point, 16 parallel, 15 point on line, 14 perpendicular, 10 horizontal, 6 centre point, 6 vertical, 5 coincident, 2 midpoint, 1 tangent, 6 other
  measures "d57" distance of L14.end L13.end
  measures "d58" distance of L17.end L18.end
  measures "d59" distance of L21.end L22.end
  measures "d60" distance of L26.end L25.end
  measures "d61" distance of L29.end L30.end
  measures "d62" distance of L36.start L36.end
  measures "d64" distance of L39.start L39.end
  measures "d65" distance of L42.end L41.end
  measures "d66" distance of L45.end L46.end
  measures "d67" diameter of A35
  measures "d68" distance of L49.start L49.end
  measures "d69" diameter of A36
  measures "d70" diameter of A38
  measures "d71" diameter of A39
extrude "Extrusion21" add sketch "Sketch18" against normal up to surface (3 mm away) contours L26 L25 L24 L4 | L28 L29 L30 L25 | L24 L32 A37 L4 | L30 L41 A39 L53 A37 L32 L24 | A37 L32 L53 L4 | L30 L37 L47 A35 L41 A37 A39 | L53 L32 L36 A32 L4 | A37 L53 L32 | L37 L38 L41 A35 L47 | A32 L36 L4 | L53 A37 L41 L47 L32 | L53 A39 L41 A37 | L36 A32 L4 | L36 L32 L47 L4 A32 | A37 L41 | L38 L32 A37 L47 A35 L41 | A35 L47 A37 L41 | L47 A37 L32 | L32 A37 L38 L46 L4 L47 | L38 A37 L32 | A6 L46 L38
extrude "Extrusion22" cut sketch "Sketch18" against normal through all contours A32 L36 L4 | L4 L36 L54 A32 | A32 A13 L54 A11 A7 | A7 L50 A5 A4 | L36 A32 L4 | L4 A32 L54 L36 | A7 A37 L7 A5 L50
extrude "Extrusion23" add sketch "Sketch18" against normal up to surface (3 mm away) contours A37 L50 A7 | A7 A32 A37 | A38 A0 L3 | A13 A32 | A32 A11 | A9 A36 | A31 L8 picked at (53.364, 415.4773) picked at (22.9339, 412.799) picked at (22.9339, 449.201) picked at (4.4806, 469.5403)
extrude "Extrusion24" cut sketch "Sketch18" against normal through all contours A38 L54 L53 | L53 L54 A38 A0 | A36 A9 L54 L49 | L49 L54 A36
sketch "Sketch19" plane through (0, 0, 0) normal (0, 0, -1) x (-1, 0, 0)
  circle A0 centre (0.5, 469.7) radius 2 projected
  line L0 (-6, 247.7791) -> (-6, -8) projected
  arc A1 (-6, -8) -> (1, -15) centre (1, -8) ccw projected
  line L1 (48.5, -15) -> (1, -15) projected
  arc A2 (48.5, -15) -> (56.1667, 76.3566) centre (48.5, 31) ccw projected
  arc A3 (54.5, 78.3286) -> (56.1667, 76.3566) centre (56.5, 78.3286) ccw projected
  line L2 (54.5, 78.3286) -> (54.5, 431) projected
  arc A4 (54.5, 431) -> (20.2113, 477) centre (6.5, 431) ccw projected
  line L3 (20.2113, 477) -> (-50.5, 477) projected
  line L4 (-50.5, 477) -> (-50.5, 247.7791) projected
  circle A5 centre (48.5, 31) radius 23.3333 projected
  circle A6 centre (23.0834, 49.4663) radius 2.1 projected
  circle A7 centre (58.2083, 60.879) radius 2.1 projected
  circle A8 centre (23.0834, 12.5337) radius 2.1 projected
  circle A9 centre (79.9167, 31) radius 2.1 projected
  circle A10 centre (58.2083, 1.121) radius 2.1 projected
  circle A11 centre (45.5, 333.7734) radius 2.25 projected
  circle A12 centre (45.5, 268.1618) radius 2.25 projected
  circle A13 centre (0.5, 333.7734) radius 2.25 projected
  circle A14 centre (0.5, 268.1618) radius 2.25 projected
  circle A15 centre (3.5, 158.6736) radius 2 projected
  circle A16 centre (42.5, -7.7) radius 2 projected
  circle A17 centre (42.5, 69.94) radius 2 projected
  circle A18 centre (42.5, 158.6736) radius 2 projected
  circle A19 centre (3.5, -7.7) radius 2 projected
  circle A20 centre (3.5, 69.94) radius 2 projected
  circle A21 centre (0.5, 392.06) radius 2 projected
  circle A22 centre (-38.5, 392.06) radius 2 projected
  circle A23 centre (-38.5, 469.7) radius 2 projected
  circle A24 centre (6.5, 431) radius 23.3333 projected
  circle A25 centre (45.5, 268.1618) radius 2.25 projected
  circle A26 centre (0.5, 268.1618) radius 2.25 projected
  line L5 (45.5, 268.1618) -> (0.5, 268.1618)
  line L6 (0.5, 268.1618) -> (-44.5, 268.1618)
  circle A27 centre (0.5, 333.7734) radius 2.25 projected
  line L7 (0.5, 333.7734) -> (-44.5, 333.7734)
  line L8 (-44.5, 333.7734) -> (-44.5, 268.1618)
  circle A28 centre (-44.5, 333.7734) radius 2
  circle A29 centre (-44.5, 268.1618) radius 2
  line L9 (-50.5, 247.7791) -> (-6, 247.7791) projected
  point P0 (0, 0)
  dimension "d81" = 45
  dimension "d82" = 45
  dimension "d83" = 4
  dimension "d84" = 4
  constraints: 8 end point, 2 centre point, 2 coincident, 2 horizontal, 1 point on line
  measures "d81" distance of L5.end L6.end
  measures "d82" distance of L7.start L7.end
  measures "d83" diameter of A28
  measures "d84" diameter of A29
extrude "Extrusion25" cut sketch "Sketch19" against normal through all contours A29 L8 L6 | L6 L8 A29 | A28 L8 L7 | L7 L8 A28
sketch "Sketch20" plane through (0, 0, 0) normal (0, 0, -1) x (-1, 0, 0)
  circle A0 centre (-44.5, 333.7734) radius 2 projected
  circle A1 centre (-44.5, 268.1618) radius 2 projected
  circle A2 centre (6.5, 431) radius 23.3333 projected
  circle A3 centre (-38.5, 469.7) radius 2 projected
  circle A4 centre (-38.5, 392.06) radius 2 projected
  circle A5 centre (0.5, 392.06) radius 2 projected
  circle A6 centre (3.5, 69.94) radius 2 projected
  circle A7 centre (3.5, -7.7) radius 2 projected
  circle A8 centre (42.5, 158.6736) radius 2 projected
  circle A9 centre (42.5, 69.94) radius 2 projected
  circle A10 centre (42.5, -7.7) radius 2 projected
  circle A11 centre (3.5, 158.6736) radius 2 projected
  circle A12 centre (0.5, 268.1618) radius 2.25 projected
  circle A13 centre (0.5, 333.7734) radius 2.25 projected
  circle A14 centre (45.5, 268.1618) radius 2.25 projected
  circle A15 centre (45.5, 333.7734) radius 2.25 projected
  circle A16 centre (58.2083, 1.121) radius 2.1 projected
  circle A17 centre (79.9167, 31) radius 2.1 projected
  circle A18 centre (23.0834, 12.5337) radius 2.1 projected
  circle A19 centre (58.2083, 60.879) radius 2.1 projected
  circle A20 centre (23.0834, 49.4663) radius 2.1 projected
  circle A21 centre (48.5, 31) radius 23.3333 projected
  arc A22 (54.5, 431) -> (20.2113, 477) centre (6.5, 431) ccw projected
  line L0 (20.2113, 477) -> (-50.5, 477) projected
  line L1 (-50.5, 477) -> (-50.5, 247.7791) projected
  line L2 (-50.5, 247.7791) -> (-6, 247.7791) projected
  line L3 (-6, 247.7791) -> (-6, -8) projected
  arc A23 (-6, -8) -> (1, -15) centre (1, -8) ccw projected
  line L4 (48.5, -15) -> (1, -15) projected
  arc A24 (48.5, -15) -> (56.1667, 76.3566) centre (48.5, 31) ccw projected
  arc A25 (54.5, 78.3286) -> (56.1667, 76.3566) centre (56.5, 78.3286) ccw projected
  line L5 (54.5, 78.3286) -> (54.5, 431) projected
  circle A26 centre (0.5, 469.7) radius 2 projected
  circle A27 centre (-44.5, 268.1618) radius 2 projected
  line L6 (-44.5, 268.1618) -> (-53.5, 268.1618)
  line L7 (-53.5, 268.1618) -> (-53.5, 333.7734)
  line L8 (-53.5, 333.7734) -> (-44.5, 333.7734)
  line L9 (-44.5, 333.7734) -> (-44.5, 268.1618)
  line L10 (-50.5, 477) -> (-50.5, 247.7791) projected
  line L11 (-53.5, 247.7791) -> (-50.5, 247.7791)
  line L12 (-50.5, 247.7791) -> (-50.5, 477)
  line L13 (-50.5, 477) -> (-53.5, 477)
  line L14 (-53.5, 477) -> (-53.5, 247.7791)
  point P0 (0, 0)
  dimension "d87" = 9
  constraints: 16 end point, 4 parallel, 2 horizontal, 2 perpendicular, 1 point on line
  measures "d87" distance of L7.end L8.end
extrude "Extrusion26" add sketch "Sketch20" against normal up to surface (3 mm away) contours L8 L14 L13 L1 | L1 L6 L7 L8 | L1 L11 L14 L6
sketch "Sketch21" plane through (0, 0, 0) normal (0, 0, -1) x (-1, 0, 0)
  circle A0 centre (0.5, 268.1618) radius 2.25 projected
  circle A1 centre (-44.5, 268.1618) radius 2 projected
  circle A2 centre (-44.5, 333.7734) radius 2 projected
  circle A3 centre (0.5, 333.7734) radius 2.25 projected
  point P0 (0, 0)
extrude "Extrusion27" add sketch "Sketch21" against normal up to surface (3 mm away)
sketch "Sketch22" plane through (0, 0, 0) normal (0, 0, -1) x (-1, 0, 0)
  line L0 (-35, 296.9804) -> (-35, 230.7)
  line L1 (-3, 296.9804) -> (-3, 230.7)
  line L2 (7, 279.9) -> (7, 230.5)
  line L3 (39, 279.9) -> (39, 230.5)
  circle A0 centre (45.5, 268.1618) radius 2.25 projected
  circle A1 centre (45.5, 268.1618) radius 2.25 construction
  line L4 (45.5, 268.1618) -> (-59.8812, 268.1618) construction
  line L5 (-53.5, 477) -> (-53.5, 247.7791) construction
  circle A2 centre (45.5, 333.7734) radius 2.25 construction
  circle A3 centre (45.5, 333.7734) radius 2.25 construction
  line L6 (45.5, 333.7734) -> (-59.8812, 333.7734) construction
  line L7 (-35, 268.1618) -> (-41.5, 268.1618)
  line L8 (-41.5, 268.1618) -> (-41.5, 333.7734)
  circle A4 centre (-41.5, 268.1618) radius 2
  circle A5 centre (-41.5, 333.7734) radius 2
  line L9 (-3, 268.1618) -> (7, 268.1618)
  line L10 (-3, 333.7734) -> (7, 333.7734)
  circle A6 centre (2, 268.1618) radius 2
  circle A7 centre (2, 333.7734) radius 2
  point P0 (0, 0)
  point P1 (-53.5, 270.3011)
  dimension "d94" = 6.5
  dimension "d95" = 4
  dimension "d96" = 4
  dimension "d97" = 4
  dimension "d98" = 4
  constraints: 20 end point, 10 point on line, 4 centre point, 4 vertical, 3 perpendicular, 2 coincident, 2 midpoint, 8 other
  measures "d94" distance of L7.start L7.end
  measures "d95" diameter of A4
  measures "d96" diameter of A5
  measures "d97" diameter of A6
  measures "d98" diameter of A7
extrude "Extrusion28" cut sketch "Sketch22" against normal through all contours A4 L8 L7 | L7 L8 A4 | A5 | A6 L9 | L9 A6 | A7 L10 | L10 A7
sketch "Sketch23" plane through (0, 0, 0) normal (0, 0, -1) x (-1, 0, 0)
  circle A0 centre (-18.9166, 412.5337) radius 2.1
  circle A1 centre (16.2083, 401.121) radius 2.1
  circle A2 centre (37.9167, 431) radius 2.1
  circle A3 centre (16.2083, 460.879) radius 2.1
  circle A4 centre (-18.9166, 449.4663) radius 2.1
  point P0 (0, 0)
  constraints: 5 centre point, 10 other
extrude "Extrusion29" cut sketch "Sketch23" against normal through all
sketch "Sketch24" plane through (0, 0, 0) normal (0, 0, -1) x (-1, 0, 0)
  arc A0 (-41.5, 275.1618) -> (-41.5, 261.1618) centre (-41.5, 268.1618) ccw
  arc A1 (-41.5, 340.7734) -> (-41.5, 326.7734) centre (-41.5, 333.7734) ccw
  line L0 (-43, 396.7333) -> (-43, 387.3867)
  line L1 (-43, 474.3733) -> (-43, 465.0267)
  circle A2 centre (37.9167, 431) radius 2.1 projected
  circle A3 centre (16.2083, 460.879) radius 2.1 projected
  circle A4 centre (16.2083, 401.121) radius 2.1 projected
  circle A5 centre (-18.9166, 449.4663) radius 2.1 projected
  circle A6 centre (-18.9166, 412.5337) radius 2.1 projected
  circle A7 centre (-41.5, 268.1618) radius 2 projected
  circle A8 centre (2, 333.7734) radius 2 projected
  circle A9 centre (-41.5, 333.7734) radius 2 projected
  circle A10 centre (2, 268.1618) radius 2 projected
  circle A11 centre (6.5, 431) radius 23.3333 projected
  circle A12 centre (-38.5, 469.7) radius 2 projected
  circle A13 centre (-38.5, 392.06) radius 2 projected
  circle A14 centre (0.5, 392.06) radius 2 projected
  circle A15 centre (3.5, 69.94) radius 2 projected
  circle A16 centre (3.5, -7.7) radius 2 projected
  circle A17 centre (42.5, 158.6736) radius 2 projected
  circle A18 centre (42.5, 69.94) radius 2 projected
  circle A19 centre (42.5, -7.7) radius 2 projected
  circle A20 centre (3.5, 158.6736) radius 2 projected
  circle A21 centre (45.5, 268.1618) radius 2.25 projected
  circle A22 centre (45.5, 333.7734) radius 2.25 projected
  circle A23 centre (58.2083, 1.121) radius 2.1 projected
  circle A24 centre (79.9167, 31) radius 2.1 projected
  circle A25 centre (23.0834, 12.5337) radius 2.1 projected
  circle A26 centre (58.2083, 60.879) radius 2.1 projected
  circle A27 centre (23.0834, 49.4663) radius 2.1 projected
  circle A28 centre (48.5, 31) radius 23.3333 projected
  arc A29 (54.5, 431) -> (20.2113, 477) centre (6.5, 431) ccw projected
  line L2 (20.2113, 477) -> (-53.5, 477) projected
  line L3 (-53.5, 477) -> (-53.5, 247.7791) projected
  line L4 (-53.5, 247.7791) -> (-6, 247.7791) projected
  line L5 (-6, 247.7791) -> (-6, -8) projected
  arc A30 (-6, -8) -> (1, -15) centre (1, -8) ccw projected
  line L6 (48.5, -15) -> (1, -15) projected
  arc A31 (48.5, -15) -> (56.1667, 76.3566) centre (48.5, 31) ccw projected
  arc A32 (54.5, 78.3286) -> (56.1667, 76.3566) centre (56.5, 78.3286) ccw projected
  line L7 (54.5, 78.3286) -> (54.5, 431) projected
  circle A33 centre (0.5, 469.7) radius 2 projected
  line L8 (-48.5, 268.1618) -> (-48.5, 247.7791)
  line L9 (-48.5, 268.1618) -> (-48.5, 477)
  line L10 (-53.5, 477) -> (20.2113, 477) projected
  point P0 (0, 0)
  constraints: 8 end point, 5 point on circle, 3 point on line, 3 vertical, 2 centre point, 1 tangent, 12 other
extrude "Extrusion30" cut sketch "Sketch24" against normal through all contours L9 L8 L4 L3 L2
fillet "Fillet9" radius 10 1 edges at (48.5, 477, 1.5)
fillet "Fillet10" radius 30 1 edges at (6, 247.7791, 1.5)
fillet "Fillet11" radius 10 1 edges at (48.5, 247.7791, 1.5)
body "Solid1"
